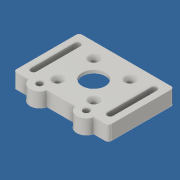
# Autodesk Inventor part: GearedStepper_RotBase
Saved by Autodesk Inventor 2016 (Build 200138000, 138)
## iProperties
Created: 2015-10-12
Part Number: GearedStepper_RotBase
Material: ABS-Kunststoff
Document SubType Name: Modeling
Designer: 4ndreas
Density: 1.06 g/cm^3
Appearance: Glatt - weiß
Author: 4ndreas
Autodesk Inventor part; units mm, degrees
ref_plane "YZ Plane" through (0, 0, 0) normal (1, 0, 0) x (0, 1, 0)
ref_plane "XZ Plane" through (0, 0, 0) normal (0, 1, 0) x (-1, 0, 0)
ref_plane "XY Plane" through (0, 0, 0) normal (0, 0, 1) x (1, 0, 0)
sketch "Skizze1" plane through (0, 0, 0) normal (0, 0, 1) x (1, 0, 0)
  circle A0 centre (0, 0) radius 4.5 projected
  line L0 (4.899, 11.5) -> (-4.899, 11.5) projected
  arc A1 (-4.899, 11.5) -> (-4.899, -11.5) centre (0, 0) ccw projected
  line L1 (-4.899, -11.5) -> (4.899, -11.5) projected
  arc A2 (4.899, -11.5) -> (4.899, 11.5) centre (0, 0) ccw projected
  arc A3 (4.899, -11.5) -> (4.899, 11.5) centre (0, 0) ccw projected
  arc A4 (-4.899, 11.5) -> (-4.899, -11.5) centre (0, 0) ccw projected
  line L2 (-4.899, -11.5) -> (4.899, -11.5) projected
  line L3 (4.899, 11.5) -> (-4.899, 11.5) projected
  circle A5 centre (0, 0) radius 21 projected
  arc A6 (-21.082, -16.7467) -> (-16.7467, -21.082) centre (0, 0) ccw projected
  line L4 (-16.7467, -21.082) -> (16.7467, -21.082) projected
  arc A7 (16.7467, -21.082) -> (21.082, -16.7467) centre (0, 0) ccw projected
  line L5 (21.082, -16.7467) -> (21.082, 16.7467) projected
  arc A8 (21.082, 16.7467) -> (16.7467, 21.082) centre (0, 0) ccw projected
  line L6 (16.7467, 21.082) -> (-16.7467, 21.082) projected
  arc A9 (-16.7467, 21.082) -> (-21.082, 16.7467) centre (0, 0) ccw projected
  line L7 (-21.082, 16.7467) -> (-21.082, -16.7467) projected
  line L8 (-32.5, -22.5) -> (32.5, -22.5)
  line L9 (32.5, -22.5) -> (32.5, 22.5)
  line L10 (32.5, 22.5) -> (-32.5, 22.5)
  line L11 (-32.5, 22.5) -> (-32.5, -22.5)
  line L12 (-32.5, -22.5) -> (32.5, 22.5) construction
  line L13 (32.5, -22.5) -> (-32.5, 22.5) construction
  arc A10 (-14.4273, -15.2596) -> (14.4273, -15.2596) centre (0, 0) ccw projected
  arc A11 (15.2596, 14.4273) -> (14.4273, 15.2596) centre (15.494, 15.494) ccw projected
  arc A12 (14.4273, -15.2596) -> (15.2596, -14.4273) centre (15.494, -15.494) ccw projected
  arc A13 (-15.2596, -14.4273) -> (-14.4273, -15.2596) centre (-15.494, -15.494) ccw projected
  arc A14 (-14.4273, 15.2596) -> (-15.2596, 14.4273) centre (-15.494, 15.494) ccw projected
  arc A15 (-15.2596, 14.4273) -> (-15.2596, -14.4273) centre (0, 0) ccw projected
  arc A16 (14.4273, 15.2596) -> (-14.4273, 15.2596) centre (0, 0) ccw projected
  arc A17 (15.2596, -14.4273) -> (15.2596, 14.4273) centre (0, 0) ccw projected
  circle A18 centre (12.3744, -12.3744) radius 1.5 projected
  circle A19 centre (12.3744, -12.3744) radius 1.5 projected
  circle A20 centre (-12.3744, -12.3744) radius 1.5 projected
  circle A21 centre (-12.3744, -12.3744) radius 1.5 projected
  circle A22 centre (-12.3744, 12.3744) radius 1.5 projected
  circle A23 centre (-12.3744, 12.3744) radius 1.5 projected
  circle A24 centre (12.3744, 12.3744) radius 1.5 projected
  circle A25 centre (12.3744, 12.3744) radius 1.5 projected
  point P0 (0, 0)
  point P1 (8.8388, 8.8388)
  point P2 (8.8388, -8.8388)
  point P3 (-8.8388, -8.8388)
  point P4 (-8.8388, 8.8388)
  dimension "d0" = 45
  dimension "d1" = 65
  constraints: 12 end point, 2 midpoint, 2 parallel, 1 horizontal, 1 perpendicular
  measures "d0" distance between parallel lines of L8 L10
  measures "d1" distance between parallel lines of L11 L9
extrude "Extrusion1" add sketch "Skizze1" against normal blind 2 contours A5 | A5 A11 | A12 A5 | A5 A14 | A13 A5 | L7 A9 L6 A8 L5 A7 L4 A6 | L11 L10 L9 L8
sketch "Skizze2" plane through (0, 0, 0) normal (0, 0, 1) x (1, 0, 0)
  circle A0 centre (0, 0) radius 8
  arc A1 (-4.899, 11.5) -> (-4.899, -11.5) centre (0, 0) ccw projected
  line L0 (-4.899, 11.5) -> (4.899, 11.5) projected
  arc A2 (4.899, -11.5) -> (4.899, 11.5) centre (0, 0) ccw projected
  line L1 (4.899, -11.5) -> (-4.899, -11.5) projected
  circle A3 centre (12.3744, 12.3744) radius 1.5 projected
  circle A4 centre (-12.3744, 12.3744) radius 1.5 projected
  circle A5 centre (-12.3744, -12.3744) radius 1.5 projected
  circle A6 centre (12.3744, -12.3744) radius 1.5 projected
  line L2 (-32.5, -22.5) -> (32.5, -22.5) projected
  line L3 (32.5, -22.5) -> (32.5, 22.5) projected
  line L4 (32.5, 22.5) -> (-32.5, 22.5) projected
  line L5 (-32.5, 22.5) -> (-32.5, -22.5) projected
  dimension "d31" = 16
  constraints: 1 centre point, 1 coincident
  measures "d31" diameter of A0
extrude "Extrusion2" add sketch "Skizze2" along normal blind 2 contours L0 A2 L1 A1 | L5 L4 L3 L2
sketch "Skizze3" plane through (0, 0, -2) normal (0, 0, -1) x (-1, 0, 0)
  circle A0 centre (0, 0) radius 21 projected
  line L0 (-32.5, -22.5) -> (32.5, -22.5) projected
  line L1 (32.5, -22.5) -> (32.5, 22.5) projected
  line L2 (32.5, 22.5) -> (-32.5, 22.5) projected
  line L3 (-32.5, 22.5) -> (-32.5, -22.5) projected
  arc A1 (4.899, -11.5) -> (4.899, 11.5) centre (0, 0) ccw projected
  line L4 (-4.899, 11.5) -> (4.899, 11.5) projected
  line L5 (4.899, -11.5) -> (-4.899, -11.5) projected
  arc A2 (-4.899, 11.5) -> (-4.899, -11.5) centre (0, 0) ccw projected
  point P0 (0, 0)
extrude "Extrusion3" add sketch "Skizze3" along normal blind 6 contours L3 L2 L1 L0
sketch "Skizze4" plane through (0, 0, 2) normal (0, 0, 1) x (1, 0, 0)
  circle A0 centre (0, 0) radius 8 projected
  line L0 (-26.25, -15) -> (-26.25, 15) construction
  line L1 (-24.25, -15) -> (-24.25, 15)
  line L2 (-28.25, 15) -> (-28.25, -15)
  arc A1 (-28.25, -15) -> (-24.25, -15) centre (-26.25, -15) ccw
  arc A2 (-24.25, 15) -> (-28.25, 15) centre (-26.25, 15) ccw
  line L3 (26.25, -15) -> (26.25, 15) construction
  line L4 (28.25, -15) -> (28.25, 15)
  line L5 (24.25, 15) -> (24.25, -15)
  arc A3 (24.25, -15) -> (28.25, -15) centre (26.25, -15) ccw
  arc A4 (28.25, 15) -> (24.25, 15) centre (26.25, 15) ccw
  line L6 (-26.25, 0) -> (26.25, 0) construction
  dimension "d10" = 4
  dimension "d11" = 30
  dimension "d32" = 52.5
  constraints: 18 end point, 8 point on circle, 8 tangent, 4 centre point, 4 parallel, 3 midpoint, 1 coincident, 1 equal radius, 1 horizontal, 1 vertical
  measures "d10" distance between parallel lines of L2 L1
  measures "d11" distance of L0.start L0.end
  measures "d32" distance of L6.start L6.end
extrude "Extrusion4" cut sketch "Skizze4" against normal through all contours A1 L2 A2 L1 | A3 L5 A4 L4
sketch "Skizze5" plane through (0, 0, -8) normal (0, 0, -1) x (-1, 0, 0)
  circle A0 centre (0, 0) radius 20
  circle A1 centre (-16, -21.1246) radius 6.5
  circle A2 centre (16, -21.1246) radius 6.5
  circle A3 centre (0, 0) radius 21 projected
  line L0 (-32.5, -22.5) -> (32.5, -22.5) projected
  line L1 (32.5, -22.5) -> (32.5, 22.5) projected
  line L2 (32.5, 22.5) -> (-32.5, 22.5) projected
  line L3 (-32.5, 22.5) -> (-32.5, -22.5) projected
  line L4 (-16, -21.1246) -> (16, -21.1246) construction
  line L5 (0, 0) -> (0, -21.1246) construction
  circle A4 centre (-16, -21.1246) radius 2.1
  circle A5 centre (16, -21.1246) radius 2.1
  dimension "d14" = 40
  dimension "d15" = 13
  dimension "d16" = 13
  dimension "d17" = 32
  dimension "d18" = 4.2
  dimension "d19" = 4.2
  constraints: 5 centre point, 4 end point, 3 coincident, 2 tangent, 1 midpoint, 1 perpendicular, 1 vertical
  measures "d14" diameter of A0
  measures "d15" diameter of A1
  measures "d16" diameter of A2
  measures "d17" distance of L4.start L4.end
  measures "d18" diameter of A4
  measures "d19" diameter of A5
extrude "Extrusion5" add sketch "Skizze5" against normal up to surface (10 mm away) contours A1 A3 | A2 A3 | A1 L0 A4 A3 | A2 L0 A5 A3 | L0 A4 A1 | L0 A5 A2
extrude "Extrusion6" cut sketch "Skizze5" against normal through all contours A4 L0 | L0 A4 | A5 L0 | L0 A5
sketch "Skizze6" plane through (0, 0, -8) normal (0, 0, -1) x (-1, 0, 0)
  circle A0 centre (-16, -21.1246) radius 2.1 projected
  circle A1 centre (16, -21.1246) radius 2.1 projected
  line L0 (22.3528, -22.5) -> (32.5, -22.5) projected
  line L1 (32.5, -22.5) -> (32.5, 22.5) projected
  line L2 (32.5, 22.5) -> (-32.5, 22.5) projected
  line L3 (-32.5, 22.5) -> (-32.5, -22.5) projected
  arc A2 (-10.091, -18.4166) -> (10.091, -18.4166) centre (0, 0) ccw projected
  line L4 (-20.0415, -21.1246) -> (-18.0207, -17.6246)
  line L5 (-18.0207, -17.6246) -> (-13.9793, -17.6246)
  line L6 (-13.9793, -17.6246) -> (-11.9585, -21.1246)
  line L7 (-11.9585, -21.1246) -> (-13.9793, -24.6246)
  line L8 (-13.9793, -24.6246) -> (-18.0207, -24.6246)
  line L9 (-18.0207, -24.6246) -> (-20.0415, -21.1246)
  line L10 (20.0415, -21.1246) -> (18.0207, -24.6246)
  line L11 (18.0207, -24.6246) -> (13.9793, -24.6246)
  line L12 (13.9793, -24.6246) -> (11.9585, -21.1246)
  line L13 (11.9585, -21.1246) -> (13.9793, -17.6246)
  line L14 (13.9793, -17.6246) -> (18.0207, -17.6246)
  line L15 (18.0207, -17.6246) -> (20.0415, -21.1246)
  line L16 (-32.5, -22.5) -> (32.5, -22.5) projected
  line L17 (-32.5, -22.5) -> (32.5, -22.5) projected
  arc A3 (-10.091, -18.4166) -> (-14.9941, -14.7029) centre (-16, -21.1246) ccw projected
  arc A4 (14.9941, -14.7029) -> (-14.9941, -14.7029) centre (0, 0) ccw projected
  arc A5 (14.9941, -14.7029) -> (10.091, -18.4166) centre (16, -21.1246) ccw projected
  line L18 (-32.5, -22.5) -> (-22.3528, -22.5) projected
  arc A6 (-22.3528, -22.5) -> (-9.6472, -22.5) centre (-16, -21.1246) ccw projected
  line L19 (-9.6472, -22.5) -> (9.6472, -22.5) projected
  arc A7 (9.6472, -22.5) -> (22.3528, -22.5) centre (16, -21.1246) ccw projected
  point P0 (0, 0)
  dimension "d24" = 7
  constraints: 24 end point, 2 coincident, 2 parallel, 1 collinear, 26 other
  measures "d24" distance between parallel lines of L8 L5
extrude "Extrusion7" cut sketch "Skizze6" against normal blind 3 contours A0 L16 L9 L4 L5 L6 L7 | A0 L16 L7 L8 L9 | L16 A1 L10 L11 L12 | L12 L13 L14 L15 L10 L16 A1
chamfer "Fase1" distance 2 angle 45 4 edges at (-13.8744, 12.3744, 2) (10.8744, 12.3744, 2) (10.8744, -12.3744, 2) (-13.8744, -12.3744, 2)
fillet "Rundung1" radius 2 4 edges at (-32.5, -22.5, -3) (32.5, -22.5, -3) (32.5, 22.5, -3) (-32.5, 22.5, -3)
sketch "Skizze7" plane through (0, 0, -8) normal (0, 0, -1) x (-1, 0, 0)
  arc A0 (32.5, 20.5) -> (30.5, 22.5) centre (30.5, 20.5) ccw projected
  line L0 (30.5, 22.5) -> (-30.5, 22.5) projected
  arc A1 (-30.5, 22.5) -> (-32.5, 20.5) centre (-30.5, 20.5) ccw projected
  line L1 (-32.5, 20.5) -> (-32.5, -20.5) projected
  arc A2 (-32.5, -20.5) -> (-30.5, -22.5) centre (-30.5, -20.5) ccw projected
  line L2 (-30.5, -22.5) -> (-22.3528, -22.5) projected
  arc A3 (-22.3528, -22.5) -> (-9.6472, -22.5) centre (-16, -21.1246) ccw projected
  line L3 (-9.6472, -22.5) -> (9.6472, -22.5) projected
  arc A4 (9.6472, -22.5) -> (22.3528, -22.5) centre (16, -21.1246) ccw projected
  line L4 (22.3528, -22.5) -> (30.5, -22.5) projected
  arc A5 (30.5, -22.5) -> (32.5, -20.5) centre (30.5, -20.5) ccw projected
  line L5 (32.5, -20.5) -> (32.5, 20.5) projected
  arc A6 (-24.25, 15) -> (-28.25, 15) centre (-26.25, 15) ccw projected
  line L6 (-24.25, 15) -> (-24.25, -15) projected
  arc A7 (-28.25, -15) -> (-24.25, -15) centre (-26.25, -15) ccw projected
  line L7 (-28.25, -15) -> (-28.25, 15) projected
  arc A8 (28.25, 15) -> (24.25, 15) centre (26.25, 15) ccw projected
  line L8 (28.25, 15) -> (28.25, -15) projected
  arc A9 (24.25, -15) -> (28.25, -15) centre (26.25, -15) ccw projected
  line L9 (24.25, -15) -> (24.25, 15) projected
  arc A10 (-10.091, -18.4166) -> (10.091, -18.4166) centre (0, 0) ccw projected
  arc A11 (-10.091, -18.4166) -> (-14.9941, -14.7029) centre (-16, -21.1246) ccw projected
  arc A12 (14.9941, -14.7029) -> (-14.9941, -14.7029) centre (0, 0) ccw projected
  arc A13 (14.9941, -14.7029) -> (10.091, -18.4166) centre (16, -21.1246) ccw projected
  line L10 (18.0207, -17.6246) -> (20.0415, -21.1246) projected
  line L11 (20.0415, -21.1246) -> (18.0207, -24.6246) projected
  line L12 (18.0207, -24.6246) -> (13.9793, -24.6246) projected
  line L13 (13.9793, -24.6246) -> (11.9585, -21.1246) projected
  line L14 (11.9585, -21.1246) -> (13.9793, -17.6246) projected
  line L15 (13.9793, -17.6246) -> (18.0207, -17.6246) projected
  line L16 (-18.0207, -24.6246) -> (-20.0415, -21.1246) projected
  line L17 (-20.0415, -21.1246) -> (-18.0207, -17.6246) projected
  line L18 (-18.0207, -17.6246) -> (-13.9793, -17.6246) projected
  line L19 (-13.9793, -17.6246) -> (-11.9585, -21.1246) projected
  line L20 (-11.9585, -21.1246) -> (-13.9793, -24.6246) projected
  line L21 (-13.9793, -24.6246) -> (-18.0207, -24.6246) projected
  circle A14 centre (0, 0) radius 21
  point P0 (0, 0)
  constraints: 1 coincident, 3 other
extrude "Extrusion8" cut sketch "Skizze7" against normal up to surface (6 mm away) contours A11 A12 A13 A10 | A14 A11 | A13 A14
